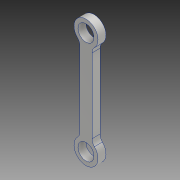
# Autodesk Inventor part: dip_pip_tendon
Saved by Autodesk Inventor 2017 SP1 (Build 210196100, 196)
## iProperties
Created: 2017-06-05
Part Number: dip_pip_tendon
Material: Generic
Document SubType Name: Modeling
Designer: Tomasz
Density: 1 g/cm^3
Appearance: Aluminum - Flat
Author: Tomasz
Autodesk Inventor part; units mm, degrees
ref_plane "YZ Plane" through (0, 0, 0) normal (1, 0, 0) x (0, 1, 0)
ref_plane "XZ Plane" through (0, 0, 0) normal (0, 1, 0) x (-1, 0, 0)
ref_plane "XY Plane" through (0, 0, 0) normal (0, 0, 1) x (1, 0, 0)
sketch "Sketch1" plane through (0, 0, 0) normal (0, 1, 0) x (-1, 0, 0)
  circle A0 centre (0, 0) radius 2
  arc A1 (2.1, -2.1424) -> (-2.1, -2.1424) centre (0, 0) ccw
  circle A2 centre (0, -25.6944) radius 2
  arc A3 (-2.1, -23.5519) -> (2.1, -23.5519) centre (0, -25.6944) ccw
  line L0 (1.5, -3.5707) -> (1.5, -22.1236)
  line L1 (-1.5, -3.5707) -> (-1.5, -22.1236)
  line L2 (0, 0) -> (0, -25.6944) construction
  arc A4 (2.1, -2.1424) -> (1.5, -3.5707) centre (3.5, -3.5707) ccw
  arc A5 (-1.5, -3.5707) -> (-2.1, -2.1424) centre (-3.5, -3.5707) ccw
  arc A6 (-2.1, -23.5519) -> (-1.5, -22.1236) centre (-3.5, -22.1236) ccw
  arc A7 (1.5, -22.1236) -> (2.1, -23.5519) centre (3.5, -22.1236) ccw
  point P0 (1.5, -2.5981)
  point P1 (-1.5, -23.0963)
  point P2 (-1.5, -2.5981)
  point P3 (1.5, -23.0963)
  dimension "d0" = 4
  dimension "d1" = 6
  dimension "d2" = 25.6944
  dimension "d3" = 4
  dimension "d4" = 6
  dimension "d5" = 3
  dimension "d6" = 2
  constraints: 16 point on circle, 8 centre point, 8 tangent, 6 end point, 4 point on line, 3 coincident, 3 equal radius, 2 vertical, 1 parallel, 1 vertical alignment, 1 other
  measures "d0" diameter of A0
  measures "d1" diameter of A1
  measures "d2" distance of A2.centre point (0, 0)
  measures "d3" diameter of A2
  measures "d4" diameter of A3
  measures "d5" distance between parallel lines of L1 L0
  measures "d6" radius of A4
extrude "Extrusion1" add sketch "Sketch1" along normal blind 2
equation "\"d2\" = length"
equation "\"d3\" = d0"
equation "\"d4\" = d1"
equation "\"length\" = 25.69436"
body "Solid1"
